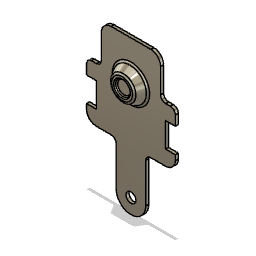
板バネプラス (Autodesk Fusion 360 design; units mm, degrees)
Autodesk Fusion 360 part; units mm, degrees
sketch "スケッチ1" plane through (0, 0, 0) normal (0, 0, 1) x (1, 0, 0)
  line L0 (4.5, 1) -> (4.5, 5)
  line L1 (-4.5, 5) -> (-4.5, 1)
  line L2 (1.5, -4.5) -> (1.5, -0.5)
  line L3 (-1.5, -4.5) -> (-1.5, -0.5)
  line L4 (-0.0005, -6) -> (0.0005, -6)
  arc A0 (-1.5, -4.5) -> (1.5, -4.5) centre (0, -4.5) ccw
  circle A1 centre (0, -4.5) radius 0.5
  line L5 (-3.5, 0) -> (-2, 0)
  line L6 (2, 0) -> (3.5, 0)
  line L7 (4.5, 1.5) -> (3.5, 1.5)
  line L8 (-4.5, 1.5) -> (-3.5, 1.5)
  arc A2 (3.5, 0) -> (4.5, 1) centre (3.5, 1) ccw
  arc A3 (-4.5, 1) -> (-3.5, 0) centre (-3.5, 1) ccw
  arc A4 (-1.5, -0.5) -> (-2, 0) centre (-2, -0.5) ccw
  arc A5 (2, 0) -> (1.5, -0.5) centre (2, -0.5) ccw
  line L9 (-2, 9.5) -> (2, 9.5)
  line L10 (3, 8.5) -> (3, 6)
  line L11 (3.5, 5.5) -> (4, 5.5)
  line L12 (-4, 5.5) -> (-3.5, 5.5)
  line L13 (-3, 6) -> (-3, 8.5)
  line L14 (-3.5, 4) -> (-3.5, 1.5)
  line L15 (-3.5, 4) -> (-4.5, 4)
  line L16 (3.5, 4) -> (3.5, 1.5)
  line L17 (3.5, 4) -> (4.5, 4)
  arc A6 (-2, 9.5) -> (-3, 8.5) centre (-2, 8.5) ccw
  arc A7 (3, 8.5) -> (2, 9.5) centre (2, 8.5) ccw
  arc A8 (-3.5, 5.5) -> (-3, 6) centre (-3.5, 6) ccw
  arc A9 (-4, 5.5) -> (-4.5, 5) centre (-4, 5) ccw
  arc A10 (3, 6) -> (3.5, 5.5) centre (3.5, 6) ccw
  arc A11 (4.5, 5) -> (4, 5.5) centre (4, 5) ccw
  circle A12 centre (0, 5.5) radius 1.2
  circle A13 centre (0, 5.5) radius 1.75
  constraint coincident A0 L4.end
  constraint coincident L1 L15.end
  constraint coincident L0 L17.end
extrude "押し出し1" add sketch "スケッチ1" along normal blind 0.3 contours L0 L1 L2 L3 A0 L5 L6 L7 L8 A2 A3 A4 A5 L9 L10 L11 L12 L13 L14 L15 L16 L17 A6 A7 A8 A9 A10 A11 | A12 | A13
ref_plane "作業平面1" through (0, 5.5, -0.9) normal (0, 0, 1) x (1, 0, 0)
sketch "スケッチ6" plane through (0, 0, -0.9) normal (0, 0, 1) x (1, 0, 0)
  circle A0 centre (0, 5.5) radius 1.2
loft "ロフト1" add profiles "スケッチ6", "スケッチ1" section 1 section 2 contours A12 | A13
fillet "フィレット1" radius 0.25 2 edges at (-1.6316, 4.8672, 0) (-1.1188, 5.0661, -0.9)
sketch "スケッチ7" plane through (0, 0, -0.9) normal (0, 0, -1) x (-1, 0, 0)
  circle A0 centre (0, 5.5) radius 1.0598
  circle A1 centre (0, 5.5) radius 0.75
  constraint concentric A0 A1
extrude "押し出し2" cut sketch "スケッチ7" against normal blind 0.2 contours A1
fillet "フィレット2" radius 0.1 2 edges at (0.6992, 5.7712, -0.7) (0.6992, 5.7712, -0.9)
move_body "移動3" bodies 1 to x (-1, 0, 0) y (0, 1, 0) z (0, 0, -1) at (0, 0, 0.3)
